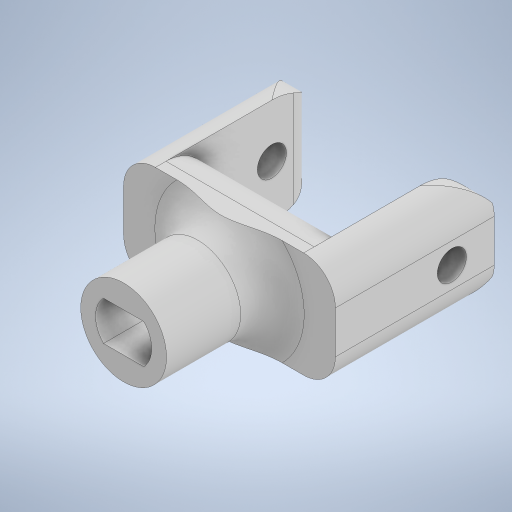
# Autodesk Inventor part: differantial
Saved by Autodesk Inventor 2023.2 (Build 272271000, 271)
## iProperties
Created: 2022-11-25
Part Number: differantial
Material: Generic
Document SubType Name: Modeling
Designer: omrfrkmll
Density: 1 g/cm^3
Appearance: Default
Author: omrfrkmll
Autodesk Inventor part; units mm, degrees
ref_plane "YZ Plane" through (0, 0, 0) normal (1, 0, 0) x (0, 1, 0)
ref_plane "XZ Plane" through (0, 0, 0) normal (0, 1, 0) x (-1, 0, 0)
ref_plane "XY Plane" through (0, 0, 0) normal (0, 0, 1) x (1, 0, 0)
sketch "Sketch1" plane through (0, 0, 0) normal (0, 0, 1) x (1, 0, 0)
  circle A0 centre (0, 0) radius 2.65
  line L0 (-2.9712, 0) -> (4.0448, 0)
  line L1 (-1.8974, 1.85) -> (1.8974, 1.85)
  line L2 (-1.8974, -1.85) -> (1.8974, -1.85)
  circle A1 centre (0, 0) radius 4.05
  dimension "d0" = 5.3
  dimension "d1" = 3.7
  dimension "d2" = 1.4
  constraints: 6 end point, 4 horizontal, 4 point on circle, 2 centre point, 1 coincident, 1 other
  measures "d0" diameter of A0
  measures "d1" distance between parallel lines of L2 L1
  measures "d2" radial gap between concentric circles of A0 A1
extrude "Extrusion1" add sketch "Sketch1" along normal blind 10 contours L1 A0 | A0 L2 | A1
sketch "Sketch2" plane through (0, 0, 0) normal (0, 0, -1) x (-1, 0, 0)
  line L0 (-7, 5) -> (7, 5)
  line L1 (10, 2) -> (10, -2)
  line L2 (7, -5) -> (-7, -5)
  line L3 (-10, -2) -> (-10, 2)
  line L4 (0, 5.5458) -> (0, -5.0999)
  line L5 (-6.6393, 0) -> (7.0922, 0)
  arc A0 (-7, 5) -> (-10, 2) centre (-7, 2) ccw
  arc A1 (10, 2) -> (7, 5) centre (7, 2) ccw
  arc A2 (7, -5) -> (10, -2) centre (7, -2) ccw
  arc A3 (-10, -2) -> (-7, -5) centre (-7, -2) ccw
  point P0 (0, 0)
  dimension "d5" = 10
  dimension "d6" = 20
  dimension "d7" = 3
  constraints: 12 end point, 8 point on circle, 8 tangent, 4 centre point, 3 equal radius, 3 horizontal, 2 parallel, 2 vertical, 1 perpendicular, 2 other
  measures "d5" distance between parallel lines of L2 L0
  measures "d6" distance between parallel lines of L3 L1
  measures "d7" radius of A0
extrude "Extrusion2" add sketch "Sketch2" along normal blind 15
sketch "Sketch3" plane through (-7, 5, 0) normal (0, 1, 0) x (1, 0, 0)
  line L0 (14, 15) -> (0, 15) projected
  line L1 (14, 0) -> (14, 15) projected
  line L2 (0, 15) -> (14, 15)
  line L3 (14, 15) -> (14, 5)
  line L4 (14, 5) -> (0, 5)
  line L5 (0, 5) -> (0, 15)
  line L6 (0, 0) -> (14, 0) projected
  point P0 (7, 0)
  dimension "d10" = 5
  constraints: 8 end point, 2 parallel, 1 horizontal, 1 perpendicular, 1 point on line
  measures "d10" distance between parallel lines of L6 L4
extrude "Extrusion3" cut sketch "Sketch3" against normal up to surface (10 mm away)
sketch "Sketch4" plane through (10, -2, 0) normal (1, 0, 0) x (0, 0, -1)
  circle A0 centre (11, 2) radius 1.375
  line L0 (15, 4) -> (15, 0) projected
  point P0 (0, 2)
  point P1 (15, 2)
  dimension "d13" = 2.75
  dimension "d14" = 4
  constraints: 1 centre point, 1 midpoint
  measures "d13" diameter of A0
  measures "d14" distance of point (15, 2) A0.centre
extrude "Extrusion4" cut sketch "Sketch4" against normal up to surface (20 mm away)
sketch "Sketch5" plane through (10, -2, 0) normal (1, 0, 0) x (0, 0, -1)
  circle A0 centre (11, 2) radius 1.375 projected
  circle A1 centre (11, 2) radius 5
  line L0 (5, 7) -> (15, 7) projected
  line L1 (11, 7) -> (15, 7)
  line L2 (15, 7) -> (15, 5)
  line L3 (15, -3) -> (15, 7) projected
  line L4 (15, -1) -> (15, -3)
  line L5 (15, -3) -> (11, -3)
  line L6 (5, -3) -> (15, -3) projected
  point P0 (0, 2)
  constraints: 8 end point, 4 point on circle, 4 point on line, 2 collinear, 2 tangent, 1 centre point, 1 coincident
extrude "Extrusion5" cut sketch "Sketch5" against normal up to surface (20 mm away) contours A1 L0 L2 | L3 L5 A1
fillet "Fillet1" radius 4 2 edges at (0, 5, -5) (0, -5, -5)
fillet "Fillet2" radius 3 1 edges at (-4.05, 0, 0)
fillet "Fillet3" radius 2 2 edges at (7, 0, -15) (-7, 0, -15)
body "Solid1"
